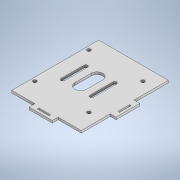
# Autodesk Inventor part: mount
Saved by Autodesk Inventor 2020 (Build 240168000, 168)
## iProperties
Created: 2019-06-18
Part Number: mount
Material: Generic
Document SubType Name: Modeling
Designer: Vivek Muskan
Density: 1 g/cm^3
Appearance: Default
Author: Vivek Muskan
Autodesk Inventor part; units mm, degrees
ref_plane "YZ Plane" through (0, 0, 0) normal (1, 0, 0) x (0, 1, 0)
ref_plane "XZ Plane" through (0, 0, 0) normal (0, 1, 0) x (-1, 0, 0)
ref_plane "XY Plane" through (0, 0, 0) normal (0, 0, 1) x (1, 0, 0)
sketch "Sketch1" plane through (0, 0, 0) normal (0, 1, 0) x (-1, 0, 0)
  circle A0 centre (0, 0) radius 5
  line L0 (0, 0) -> (12.5, 0)
  line L1 (12.5, 10) -> (12.5, -10) construction
  line L2 (11, 10) -> (11, -10)
  line L3 (14, -10) -> (14, 10)
  arc A1 (14, 10) -> (11, 10) centre (12.5, 10) ccw
  arc A2 (11, -10) -> (14, -10) centre (12.5, -10) ccw
  circle A3 centre (0, 0) radius 24
  line L4 (0, 0) -> (-33.5, 0)
  line L5 (0, 0) -> (0, 43.5)
  line L6 (-33.5, 0) -> (-33.5, 40)
  line L7 (-33.5, 40) -> (26.5, 40)
  line L8 (26.5, 40) -> (26.5, -35)
  line L9 (26.5, -35) -> (-33.5, -35)
  line L10 (-33.5, -35) -> (-33.5, 0)
  line L11 (-33.5, 40) -> (-13.5, 40)
  line L12 (-13.5, 40) -> (6.5, 40)
  line L13 (6.5, 40) -> (6.5, 45)
  line L14 (6.5, 45) -> (-13.5, 45)
  line L15 (-13.5, 45) -> (-13.5, 40)
  line L16 (-33.5, 40) -> (-33.5, 15)
  line L17 (-33.5, 15) -> (-38.5, 15)
  line L18 (-38.5, 15) -> (-38.5, -5.425)
  line L19 (-38.5, -5.425) -> (-33.5, -5.425)
  line L20 (-33.5, -5.425) -> (-33.5, 15)
  line L21 (-33.5, 15) -> (-35, 15)
  line L22 (-35, 15) -> (-35, 10)
  line L23 (-35, 10) -> (-36.5, 10)
  line L24 (-36.5, 10) -> (-36.5, 0)
  line L25 (-36.5, 0) -> (-35, 0)
  line L26 (-35, 0) -> (-35, 10)
  line L27 (6.5, 40) -> (1.5, 40)
  line L28 (1.5, 40) -> (1.5, 41.5)
  line L29 (1.5, 41.5) -> (-8.5, 41.5)
  line L30 (-8.5, 41.5) -> (-8.5, 43)
  line L31 (-8.5, 43) -> (1.5, 43)
  line L32 (1.5, 43) -> (1.5, 41.5)
  line L33 (0, 0) -> (23.3345, -23.3345)
  line L34 (0, 0) -> (33, 0) construction
  circle A4 centre (23.3345, -23.3345) radius 1.5
  circle A5 centre (23.3345, 23.3345) radius 1.5
  circle A6 centre (-23.3345, 23.3345) radius 1.5
  circle A7 centre (-23.3345, -23.3345) radius 1.5
  line L35 (-11, 10) -> (-11, -10)
  line L36 (-14, -10) -> (-14, 10)
  arc A8 (-11, 10) -> (-14, 10) centre (-12.5, 10) ccw
  arc A9 (-14, -10) -> (-11, -10) centre (-12.5, -10) ccw
  point P0 (6.5, 40)
  dimension "d0" = 10
  dimension "d1" = 12.5
  dimension "d2" = 10
  dimension "d3" = 3
  dimension "d6" = 48
  dimension "d7" = 33.5
  dimension "d8" = 43.5
  dimension "d9" = 60
  dimension "d10" = 75
  dimension "d11" = 20
  dimension "d12" = 20
  dimension "d13" = 5
  dimension "d14" = 25
  dimension "d15" = 5
  dimension "d16" = 1.5
  dimension "d17" = 5
  dimension "d18" = 1.5
  dimension "d19" = 10
  dimension "d20" = 5
  dimension "d21" = 1.5
  dimension "d22" = 10
  dimension "d23" = 1.5
  dimension "d24" = 33
  dimension "d25" = 45
  dimension "d26" = 3
  dimension "d29" = 360
  constraints: 76 end point, 10 centre point, 9 parallel, 9 perpendicular, 8 point on circle, 6 horizontal, 6 symmetric about line, 5 point on line, 4 tangent, 4 vertical, 3 coincident, 1 equal length, 1 midpoint, 11 other
  measures "d0" diameter of A0
  measures "d1" distance of L0.start L0.end
  measures "d2" distance of L0.end L1.end
  measures "d3" diameter of A2
  measures "d6" diameter of A3
  measures "d7" distance of L4.start L4.end
  measures "d8" distance of L4.start L5.end
  measures "d9" distance of L6.end L7.end
  measures "d10" distance of L7.end L8.end
  measures "d11" distance of L6.end L11.end
  measures "d12" distance of L14.end L13.end
  measures "d13" distance of L13.end L12.end
  measures "d14" distance of L6.end L16.end
  measures "d15" distance of L19.end L18.end
  measures "d16" distance of L16.end L21.end
  measures "d17" distance of L21.end L22.end
  measures "d18" distance of L25.end L24.end
  measures "d19" distance of L24.end L23.end
  measures "d20" distance of L12.end L27.end
  measures "d21" distance of L27.end L28.end
  measures "d22" distance of L30.end L31.end
  measures "d23" distance of L29.end L30.end
  measures "d24" distance of L4.start L33.end
  measures "d25" angle of L33 L34
  measures "d26" diameter of A4
extrude "Extrusion1" add sketch "Sketch1" along normal blind 2 contours A0 L5 A3 L33 | A0 L4 L35 A8 L36 A3 L5 | L33 A3 L4 L36 A9 L35 A0 | L5 L7 L8 L9 L10 L4 A3 | A3 L4 L6 L7 L5 | L7 L15 L14 L13 L28 L32 L31 L30 L29 L5 | L5 L29 L28 L7 | L26 L25 L24 L23 | L10 L19 L18 L17 L6
extrude "Extrusion2" cut sketch "Sketch1" along normal blind 2 contours L26 L25 L24 L23
sketch "Sketch2" plane through (0, 2, 0) normal (0, 1, 0) x (1, 0, 0)
  line L0 (0, -7) -> (0, 7) construction
  line L1 (5, -7) -> (5, 7)
  line L2 (-5, 7) -> (-5, -7)
  arc A0 (-5, -7) -> (5, -7) centre (0, -7) ccw
  arc A1 (5, 7) -> (-5, 7) centre (0, 7) ccw
  point P0 (0, 0)
  dimension "d35" = 7
  dimension "d36" = 10
  constraints: 8 end point, 4 point on circle, 4 tangent, 2 centre point, 1 midpoint, 1 parallel, 1 vertical
  measures "d35" distance of point (0, 0) L0.end
  measures "d36" diameter of A1
extrude "Extrusion3" cut sketch "Sketch2" against normal blind 10
body "Solid1"
